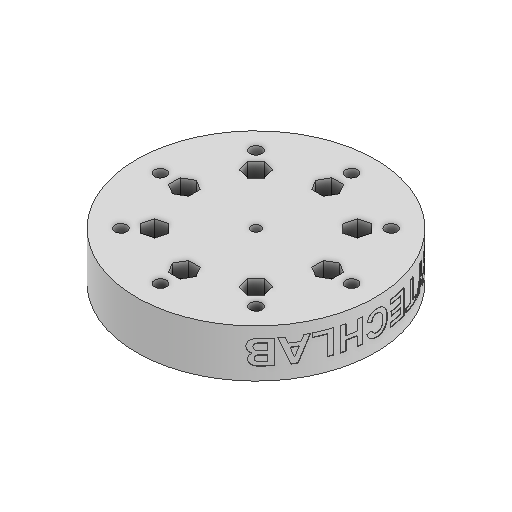
# Autodesk Inventor part: 3DP_ASA_Cone_and_Disc_Mount
Saved by Autodesk Inventor 2026.1 (Build 301233000, 233)
## iProperties
Created: 2025-06-20
Part Number: 3DP_ASA_Cone_and_Disc_Mount
Material: Generic
Document SubType Name: Modeling
Designer: User
Density: 1 g/cm^3
Appearance: Default
Author: User
Autodesk Inventor part; units mm, degrees
ref_plane "XZ Plane" through (0, 0, 0) normal (0, 1, 0) x (-1, 0, 0)
ref_plane "XY Plane" through (0, 0, 0) normal (0, 0, 1) x (1, 0, 0)
sketch "Sketch1" plane through (0, 0, 0) normal (0, 1, 0) x (-1, 0, 0)
  circle A0 centre (0, 0) radius 50
  line L0 (0, 50) -> (0, -50)
  point P0 (0, 40)
  point P1 (-28.2843, 28.2843)
  point P2 (-40, 0)
  point P3 (-28.2843, -28.2843)
  point P4 (0, -40)
  point P5 (28.2843, -28.2843)
  point P6 (40, 0)
  point P7 (28.2843, 28.2843)
  point P8 (0, 30)
  point P9 (-21.2132, 21.2132)
  point P10 (-30, 0)
  point P11 (-21.2132, -21.2132)
  point P12 (0, -30)
  point P13 (21.2132, -21.2132)
  point P14 (30, 0)
  point P15 (21.2132, 21.2132)
  dimension "d0" = 100
  dimension "d1" = 40
  dimension "d4" = 360
  dimension "d15" = 30
  dimension "d18" = 360
  constraints: 2 end point, 2 point on circle, 2 point on line, 1 centre point, 1 coincident, 1 midpoint, 1 vertical, 18 other
  measures "d0" diameter of A0
  measures "d1" distance of point (0, 0) point (0, 40)
  measures "d15" distance of point (0, 0) point (0, 30)
extrude "Extrusion1" add sketch "Sketch1" along normal blind 20
hole "Hole2" at (0, 0, 40) at (28.2843, 0, 28.2843) at (40, 0, 0) at (28.2843, 0, -28.2843) at (0, 0, -40) at (-28.2843, 0, -28.2843) at (-40, 0, 0) at (-28.2843, 0, 28.2843) at (0, 0, 30) at (21.2132, 0, 21.2132) at (30, 0, 0) at (21.2132, 0, -21.2132) at (0, 0, -30) at (-21.2132, 0, -21.2132) at (-30, 0, 0) at (-21.2132, 0, 21.2132) direction (0, 1, 0) diameter 5 end through all
sketch "Sketch2" plane through (0, 20, 0) normal (0, 1, 0) x (1, 0, 0)
  circle A0 centre (-21.2132, -21.2132) radius 2.5 projected
  circle A1 centre (-30, 0) radius 2.5 projected
  circle A2 centre (-21.2132, 21.2132) radius 2.5 projected
  circle A3 centre (0, 30) radius 2.5 projected
  circle A4 centre (21.2132, 21.2132) radius 2.5 projected
  circle A5 centre (30, 0) radius 2.5 projected
  circle A6 centre (21.2132, -21.2132) radius 2.5 projected
  circle A7 centre (0, -30) radius 2.5 projected
  circle A8 centre (-28.2843, -28.2843) radius 2.5 projected
  circle A9 centre (-40, 0) radius 2.5 projected
  circle A10 centre (-28.2843, 28.2843) radius 2.5 projected
  circle A11 centre (0, 40) radius 2.5 projected
  circle A12 centre (28.2843, 28.2843) radius 2.5 projected
  circle A13 centre (40, 0) radius 2.5 projected
  circle A14 centre (28.2843, -28.2843) radius 2.5 projected
  circle A15 centre (0, -40) radius 2.5 projected
  circle A16 centre (0, 0) radius 50 projected
  line L0 (-2.4537, -34.25) -> (-4.9075, -30)
  line L1 (-4.9075, -30) -> (-2.4537, -25.75)
  line L2 (-2.4537, -25.75) -> (2.4537, -25.75)
  line L3 (2.4537, -25.75) -> (4.9075, -30)
  line L4 (4.9075, -30) -> (2.4537, -34.25)
  line L5 (2.4537, -34.25) -> (-2.4537, -34.25)
  line L6 (16.4729, -19.9431) -> (19.9431, -16.4729)
  line L7 (19.9431, -16.4729) -> (24.6833, -17.7431)
  line L8 (17.7431, -24.6833) -> (16.4729, -19.9431)
  line L9 (24.6833, -17.7431) -> (25.9535, -22.4834)
  line L10 (25.9535, -22.4834) -> (22.4834, -25.9535)
  line L11 (22.4834, -25.9535) -> (17.7431, -24.6833)
  line L12 (25.75, -2.4537) -> (25.75, 2.4537)
  line L13 (25.75, 2.4537) -> (30, 4.9075)
  line L14 (30, -4.9075) -> (25.75, -2.4537)
  line L15 (30, 4.9075) -> (34.25, 2.4537)
  line L16 (34.25, 2.4537) -> (34.25, -2.4537)
  line L17 (34.25, -2.4537) -> (30, -4.9075)
  line L18 (19.9431, 16.4729) -> (16.4729, 19.9431)
  line L19 (16.4729, 19.9431) -> (17.7431, 24.6833)
  line L20 (24.6833, 17.7431) -> (19.9431, 16.4729)
  line L21 (17.7431, 24.6833) -> (22.4834, 25.9535)
  line L22 (22.4834, 25.9535) -> (25.9535, 22.4834)
  line L23 (25.9535, 22.4834) -> (24.6833, 17.7431)
  line L24 (2.4537, 25.75) -> (-2.4537, 25.75)
  line L25 (-2.4537, 25.75) -> (-4.9075, 30)
  line L26 (4.9075, 30) -> (2.4537, 25.75)
  line L27 (-4.9075, 30) -> (-2.4537, 34.25)
  line L28 (-2.4537, 34.25) -> (2.4537, 34.25)
  line L29 (2.4537, 34.25) -> (4.9075, 30)
  line L30 (-16.4729, 19.9431) -> (-19.9431, 16.4729)
  line L31 (-19.9431, 16.4729) -> (-24.6833, 17.7431)
  line L32 (-17.7431, 24.6833) -> (-16.4729, 19.9431)
  line L33 (-24.6833, 17.7431) -> (-25.9535, 22.4834)
  line L34 (-25.9535, 22.4834) -> (-22.4834, 25.9535)
  line L35 (-22.4834, 25.9535) -> (-17.7431, 24.6833)
  line L36 (-25.75, 2.4537) -> (-25.75, -2.4537)
  line L37 (-25.75, -2.4537) -> (-30, -4.9075)
  line L38 (-30, 4.9075) -> (-25.75, 2.4537)
  line L39 (-30, -4.9075) -> (-34.25, -2.4537)
  line L40 (-34.25, -2.4537) -> (-34.25, 2.4537)
  line L41 (-34.25, 2.4537) -> (-30, 4.9075)
  line L42 (-19.9431, -16.4729) -> (-16.4729, -19.9431)
  line L43 (-16.4729, -19.9431) -> (-17.7431, -24.6833)
  line L44 (-24.6833, -17.7431) -> (-19.9431, -16.4729)
  line L45 (-17.7431, -24.6833) -> (-22.4834, -25.9535)
  line L46 (-22.4834, -25.9535) -> (-25.9535, -22.4834)
  line L47 (-25.9535, -22.4834) -> (-24.6833, -17.7431)
  point P0 (30, 0)
  point P1 (21.2132, 21.2132)
  point P2 (0, 30)
  point P3 (-21.2132, 21.2132)
  point P4 (-30, 0)
  dimension "d27" = 8.5
  dimension "d30" = 360
  constraints: 96 end point, 1 coincident, 118 other
  measures "d27" distance between parallel lines of L2 L5
extrude "Extrusion2" cut sketch "Sketch2" against normal blind 12.5 contours L0 L1 L2 L3 L4 L5 | L6 L7 L9 L10 L11 L8 | L12 L13 L15 L16 L17 L14 | L18 L19 L21 L22 L23 L20 | L24 L25 L27 L28 L29 L26 | L30 L31 L33 L34 L35 L32 | L36 L37 L39 L40 L41 L38 | L42 L43 L45 L46 L47 L44
sketch "Sketch3" plane through (0, 0, 0) normal (0, -1, 0) x (1, 0, 0)
  circle A0 centre (-21.2132, 21.2132) radius 2.5 projected
  circle A1 centre (-30, 0) radius 2.5 projected
  circle A2 centre (-21.2132, -21.2132) radius 2.5 projected
  circle A3 centre (0, -30) radius 2.5 projected
  circle A4 centre (21.2132, -21.2132) radius 2.5 projected
  circle A5 centre (30, 0) radius 2.5 projected
  circle A6 centre (21.2132, 21.2132) radius 2.5 projected
  circle A7 centre (0, 30) radius 2.5 projected
  circle A8 centre (-28.2843, 28.2843) radius 2.5 projected
  circle A9 centre (-40, 0) radius 2.5 projected
  circle A10 centre (-28.2843, -28.2843) radius 2.5 projected
  circle A11 centre (0, -40) radius 2.5 projected
  circle A12 centre (28.2843, -28.2843) radius 2.5 projected
  circle A13 centre (40, 0) radius 2.5 projected
  circle A14 centre (28.2843, 28.2843) radius 2.5 projected
  circle A15 centre (0, 40) radius 2.5 projected
  circle A16 centre (0, 0) radius 50 projected
  line L0 (-35.75, -2.4537) -> (-40, -4.9075)
  line L1 (-40, -4.9075) -> (-44.25, -2.4537)
  line L2 (-44.25, -2.4537) -> (-44.25, 2.4537)
  line L3 (-44.25, 2.4537) -> (-40, 4.9075)
  line L4 (-40, 4.9075) -> (-35.75, 2.4537)
  line L5 (-35.75, 2.4537) -> (-35.75, -2.4537)
  line L6 (-27.0141, -23.544) -> (-23.544, -27.0141)
  line L7 (-31.7544, -24.8142) -> (-27.0141, -23.544)
  line L8 (-33.0245, -29.5544) -> (-31.7544, -24.8142)
  line L9 (-23.544, -27.0141) -> (-24.8142, -31.7544)
  line L10 (-29.5544, -33.0245) -> (-33.0245, -29.5544)
  line L11 (-24.8142, -31.7544) -> (-29.5544, -33.0245)
  line L12 (-2.4537, -35.75) -> (2.4537, -35.75)
  line L13 (-4.9075, -40) -> (-2.4537, -35.75)
  line L14 (-2.4537, -44.25) -> (-4.9075, -40)
  line L15 (2.4537, -35.75) -> (4.9075, -40)
  line L16 (2.4537, -44.25) -> (-2.4537, -44.25)
  line L17 (4.9075, -40) -> (2.4537, -44.25)
  line L18 (23.544, -27.0141) -> (27.0141, -23.544)
  line L19 (24.8142, -31.7544) -> (23.544, -27.0141)
  line L20 (29.5544, -33.0245) -> (24.8142, -31.7544)
  line L21 (27.0141, -23.544) -> (31.7544, -24.8142)
  line L22 (33.0245, -29.5544) -> (29.5544, -33.0245)
  line L23 (31.7544, -24.8142) -> (33.0245, -29.5544)
  line L24 (35.75, -2.4537) -> (35.75, 2.4537)
  line L25 (40, -4.9075) -> (35.75, -2.4537)
  line L26 (44.25, -2.4537) -> (40, -4.9075)
  line L27 (35.75, 2.4537) -> (40, 4.9075)
  line L28 (44.25, 2.4537) -> (44.25, -2.4537)
  line L29 (40, 4.9075) -> (44.25, 2.4537)
  line L30 (27.0141, 23.544) -> (23.544, 27.0141)
  line L31 (31.7544, 24.8142) -> (27.0141, 23.544)
  line L32 (33.0245, 29.5544) -> (31.7544, 24.8142)
  line L33 (23.544, 27.0141) -> (24.8142, 31.7544)
  line L34 (29.5544, 33.0245) -> (33.0245, 29.5544)
  line L35 (24.8142, 31.7544) -> (29.5544, 33.0245)
  line L36 (2.4537, 35.75) -> (-2.4537, 35.75)
  line L37 (4.9075, 40) -> (2.4537, 35.75)
  line L38 (2.4537, 44.25) -> (4.9075, 40)
  line L39 (-2.4537, 35.75) -> (-4.9075, 40)
  line L40 (-2.4537, 44.25) -> (2.4537, 44.25)
  line L41 (-4.9075, 40) -> (-2.4537, 44.25)
  line L42 (-23.544, 27.0141) -> (-27.0141, 23.544)
  line L43 (-24.8142, 31.7544) -> (-23.544, 27.0141)
  line L44 (-29.5544, 33.0245) -> (-24.8142, 31.7544)
  line L45 (-27.0141, 23.544) -> (-31.7544, 24.8142)
  line L46 (-33.0245, 29.5544) -> (-29.5544, 33.0245)
  line L47 (-31.7544, 24.8142) -> (-33.0245, 29.5544)
  point P0 (0, -40)
  point P1 (-28.2843, 28.2843)
  dimension "d34" = 8.5
  dimension "d37" = 360
  constraints: 96 end point, 1 coincident, 118 other
  measures "d34" distance between parallel lines of L2 L5
extrude "Extrusion3" cut sketch "Sketch3" against normal blind 12.5 contours A8 | A10 | L0 L1 L2 L3 L4 L5 | L6 L9 L11 L10 L8 L7 | L12 L15 L17 L16 L14 L13 | L18 L21 L23 L22 L20 L19 | L24 L27 L29 L28 L26 L25 | L30 L33 L35 L34 L32 L31 | L36 L39 L41 L40 L38 L37 | L42 L45 L47 L46 L44 L43
ref_plane "Work Plane1" through (50, 0, 0) normal (1, 0, 0) x (0, 1, 0)
sketch "Sketch4" plane through (50, 0, 0) normal (1, 0, 0) x (0, 1, 0)
  line L0 (5.2475, -38.8454) -> (5.2475, 38.603) construction
  line L1 (5.2475, 38.603) -> (21.5172, 38.603) construction
  line L2 (21.5172, 38.603) -> (21.5172, -38.8454) construction
  line L3 (21.5172, -38.8454) -> (5.2475, -38.8454) construction
  line L4 (5.4152, -42.1867) -> (5.4152, -38.1852)
  spline S0 degree 2 poles (5.4152, -38.1852) (5.4152, -36.9962) (5.6134, -35.83) (6.2384, -34.9078) (7.2826, -34.2904) (7.9304, -34.2904) knots 0 0 0 1 2 3 4 4 4
  spline S1 degree 2 poles (7.9304, -34.2904) (8.6316, -34.2904) (9.7978, -35.045) (10.0951, -35.6928) knots 0 0 0 1 2 2 2
  spline S2 degree 2 poles (10.0951, -35.6928) (10.3618, -34.7782) (11.6423, -33.8026) (12.5112, -33.8026) knots 0 0 0 1 2 2 2
  spline S3 degree 2 poles (12.5112, -33.8026) (13.1972, -33.8026) (14.4853, -34.4352) (15.2551, -35.5404) (15.3466, -36.3407) knots 0 0 0 1 2 3 3 3
  spline S4 degree 2 poles (15.3466, -36.3407) (15.3999, -36.8514) (15.4152, -38.7797) knots 0 0 0 1 1 1
  line L5 (15.4152, -38.7797) -> (15.4152, -42.1867)
  line L6 (15.4152, -42.1867) -> (5.4152, -42.1867)
  line L7 (11.0478, -40.1669) -> (13.7231, -40.1669)
  line L8 (13.7231, -40.1669) -> (13.7231, -38.2919)
  spline S5 degree 2 poles (13.7231, -38.2919) (13.7231, -37.1944) (13.6621, -36.9047) knots 0 0 0 1 1 1
  spline S6 degree 2 poles (13.6621, -36.9047) (13.5783, -36.455) (12.9457, -35.8834) (12.4121, -35.8834) knots 0 0 0 1 2 2 2
  spline S7 degree 2 poles (12.4121, -35.8834) (11.9624, -35.8834) (11.3374, -36.3178) (11.0478, -37.1486) (11.0478, -38.5282) knots 0 0 0 1 2 3 3 3
  line L9 (11.0478, -38.5282) -> (11.0478, -40.1669)
  line L10 (7.0768, -40.1669) -> (9.3862, -40.1669)
  line L11 (9.3862, -40.1669) -> (9.3862, -38.8407)
  spline S8 degree 2 poles (9.3862, -38.8407) (9.3862, -37.6593) (9.3557, -37.3697) knots 0 0 0 1 1 1
  spline S9 degree 2 poles (9.3557, -37.3697) (9.2871, -36.8514) (8.7002, -36.2569) (8.2124, -36.2569) knots 0 0 0 1 2 2 2
  spline S10 degree 2 poles (8.2124, -36.2569) (7.7475, -36.2569) (7.1759, -36.7675) (7.1073, -37.2782) knots 0 0 0 1 2 2 2
  spline S11 degree 2 poles (7.1073, -37.2782) (7.0768, -37.5755) (7.0768, -39.0084) knots 0 0 0 1 1 1
  line L12 (7.0768, -39.0084) -> (7.0768, -40.1669)
  line L13 (15.4152, -29.4733) -> (11.2079, -29.4733)
  line L14 (11.2079, -29.4733) -> (5.4152, -33.1319)
  line L15 (5.4152, -33.1319) -> (5.4152, -30.7691)
  line L16 (5.4152, -30.7691) -> (9.3786, -28.4062)
  line L17 (9.3786, -28.4062) -> (5.4152, -26.1044)
  line L18 (5.4152, -26.1044) -> (5.4152, -23.7721)
  line L19 (5.4152, -23.7721) -> (11.2231, -27.4535)
  line L20 (11.2231, -27.4535) -> (15.4152, -27.4535)
  line L21 (15.4152, -27.4535) -> (15.4152, -29.4733)
  line L22 (15.4152, -20.5251) -> (7.1073, -20.5251)
  line L23 (7.1073, -20.5251) -> (7.1073, -23.4901)
  line L24 (7.1073, -23.4901) -> (5.4152, -23.4901)
  line L25 (5.4152, -23.4901) -> (5.4152, -15.548)
  line L26 (5.4152, -15.548) -> (7.1073, -15.548)
  line L27 (7.1073, -15.548) -> (7.1073, -18.5053)
  line L28 (7.1073, -18.5053) -> (15.4152, -18.5053)
  line L29 (15.4152, -18.5053) -> (15.4152, -20.5251)
  line L30 (15.4152, -14.237) -> (5.4152, -14.237)
  line L31 (5.4152, -14.237) -> (5.4152, -6.8209)
  line L32 (5.4152, -6.8209) -> (7.1073, -6.8209)
  line L33 (7.1073, -6.8209) -> (7.1073, -12.2172)
  line L34 (7.1073, -12.2172) -> (9.3252, -12.2172)
  line L35 (9.3252, -12.2172) -> (9.3252, -7.1944)
  line L36 (9.3252, -7.1944) -> (11.0173, -7.1944)
  line L37 (11.0173, -7.1944) -> (11.0173, -12.2172)
  line L38 (11.0173, -12.2172) -> (13.7231, -12.2172)
  line L39 (13.7231, -12.2172) -> (13.7231, -6.6303)
  line L40 (13.7231, -6.6303) -> (15.4152, -6.6303)
  line L41 (15.4152, -6.6303) -> (15.4152, -14.237)
  line L42 (11.7338, 1.4794) -> (12.3512, 3.4383)
  spline S12 degree 2 poles (12.3512, 3.4383) (13.9899, 2.9886) (15.5829, 0.8925) (15.5829, -0.7157) knots 0 0 0 1 2 2 2
  spline S13 degree 2 poles (15.5829, -0.7157) (15.5829, -2.705) (12.8618, -5.2736) (10.5066, -5.2736) knots 0 0 0 1 2 2 2
  spline S14 degree 2 poles (10.5066, -5.2736) (8.0066, -5.2736) (5.2475, -2.6974) (5.2475, -0.5937) knots 0 0 0 1 2 2 2
  spline S15 degree 2 poles (5.2475, -0.5937) (5.2475, 1.2355) (6.3298, 2.3864) knots 0 0 0 1 1 1
  spline S16 degree 2 poles (6.3298, 2.3864) (6.9701, 3.0648) (8.1667, 3.4078) knots 0 0 0 1 1 1
  line L43 (8.1667, 3.4078) -> (8.6469, 1.4108)
  spline S17 degree 2 poles (8.6469, 1.4108) (7.8694, 1.2355) (6.9701, 0.1075) (6.9701, -0.6928) knots 0 0 0 1 2 2 2
  spline S18 degree 2 poles (6.9701, -0.6928) (6.9701, -1.8056) (8.563, -3.1928) (10.3542, -3.1928) knots 0 0 0 1 2 2 2
  spline S19 degree 2 poles (10.3542, -3.1928) (12.2521, -3.1928) (13.8603, -1.8285) (13.8603, -0.7386) knots 0 0 0 1 2 2 2
  spline S20 degree 2 poles (13.8603, -0.7386) (13.8603, 0.0694) (12.8313, 1.2279) (11.7338, 1.4794) knots 0 0 0 1 2 2 2
  line L44 (15.4152, 5.1761) -> (5.4152, 5.1761)
  line L45 (5.4152, 5.1761) -> (5.4152, 7.1959)
  line L46 (5.4152, 7.1959) -> (9.3481, 7.1959)
  line L47 (9.3481, 7.1959) -> (9.3481, 11.1517)
  line L48 (9.3481, 11.1517) -> (5.4152, 11.1517)
  line L49 (5.4152, 11.1517) -> (5.4152, 13.1715)
  line L50 (5.4152, 13.1715) -> (15.4152, 13.1715)
  line L51 (15.4152, 13.1715) -> (15.4152, 11.1517)
  line L52 (15.4152, 11.1517) -> (11.0402, 11.1517)
  line L53 (11.0402, 11.1517) -> (11.0402, 7.1959)
  line L54 (11.0402, 7.1959) -> (15.4152, 7.1959)
  line L55 (15.4152, 7.1959) -> (15.4152, 5.1761)
  line L56 (15.4152, 15.3209) -> (5.499, 15.3209)
  line L57 (5.499, 15.3209) -> (5.499, 17.3407)
  line L58 (5.499, 17.3407) -> (13.7231, 17.3407)
  line L59 (13.7231, 17.3407) -> (13.7231, 22.3636)
  line L60 (13.7231, 22.3636) -> (15.4152, 22.3636)
  line L61 (15.4152, 22.3636) -> (15.4152, 15.3209)
  line L62 (15.4152, 32.8133) -> (15.4152, 30.6181)
  line L63 (15.4152, 30.6181) -> (13.1438, 29.7492)
  line L64 (13.1438, 29.7492) -> (13.1438, 25.7553)
  line L65 (13.1438, 25.7553) -> (15.4152, 24.9245)
  line L66 (15.4152, 24.9245) -> (15.4152, 22.7828)
  line L67 (15.4152, 22.7828) -> (5.4152, 26.67)
  line L68 (5.4152, 26.67) -> (5.4152, 28.8194)
  line L69 (5.4152, 28.8194) -> (15.4152, 32.8133)
  line L70 (11.4518, 29.1014) -> (7.7475, 27.7218)
  line L71 (7.7475, 27.7218) -> (11.4518, 26.3651)
  line L72 (11.4518, 26.3651) -> (11.4518, 29.1014)
  line L73 (5.4152, 33.8956) -> (5.4152, 37.8971)
  spline S21 degree 2 poles (5.4152, 37.8971) (5.4152, 39.0861) (5.6134, 40.2523) (6.2384, 41.1745) (7.2826, 41.7919) (7.9304, 41.7919) knots 0 0 0 1 2 3 4 4 4
  spline S22 degree 2 poles (7.9304, 41.7919) (8.6316, 41.7919) (9.7978, 41.0374) (10.0951, 40.3895) knots 0 0 0 1 2 2 2
  spline S23 degree 2 poles (10.0951, 40.3895) (10.3618, 41.3041) (11.6423, 42.2797) (12.5112, 42.2797) knots 0 0 0 1 2 2 2
  spline S24 degree 2 poles (12.5112, 42.2797) (13.1972, 42.2797) (14.4853, 41.6471) (15.2551, 40.5419) (15.3466, 39.7416) knots 0 0 0 1 2 3 3 3
  spline S25 degree 2 poles (15.3466, 39.7416) (15.3999, 39.2309) (15.4152, 37.3026) knots 0 0 0 1 1 1
  line L74 (15.4152, 37.3026) -> (15.4152, 33.8956)
  line L75 (15.4152, 33.8956) -> (5.4152, 33.8956)
  line L76 (11.0478, 35.9154) -> (13.7231, 35.9154)
  line L77 (13.7231, 35.9154) -> (13.7231, 37.7904)
  spline S26 degree 2 poles (13.7231, 37.7904) (13.7231, 38.888) (13.6621, 39.1776) knots 0 0 0 1 1 1
  spline S27 degree 2 poles (13.6621, 39.1776) (13.5783, 39.6273) (12.9457, 40.1989) (12.4121, 40.1989) knots 0 0 0 1 2 2 2
  spline S28 degree 2 poles (12.4121, 40.1989) (11.9624, 40.1989) (11.3374, 39.7645) (11.0478, 38.9337) (11.0478, 37.5541) knots 0 0 0 1 2 3 3 3
  line L78 (11.0478, 37.5541) -> (11.0478, 35.9154)
  line L79 (7.0768, 35.9154) -> (9.3862, 35.9154)
  line L80 (9.3862, 35.9154) -> (9.3862, 37.2416)
  spline S29 degree 2 poles (9.3862, 37.2416) (9.3862, 38.423) (9.3557, 38.7127) knots 0 0 0 1 1 1
  spline S30 degree 2 poles (9.3557, 38.7127) (9.2871, 39.2309) (8.7002, 39.8255) (8.2124, 39.8255) knots 0 0 0 1 2 2 2
  spline S31 degree 2 poles (8.2124, 39.8255) (7.7475, 39.8255) (7.1759, 39.3148) (7.1073, 38.8041) knots 0 0 0 1 2 2 2
  spline S32 degree 2 poles (7.1073, 38.8041) (7.0768, 38.5069) (7.0768, 37.0739) knots 0 0 0 1 1 1
  line L81 (7.0768, 37.0739) -> (7.0768, 35.9154)
  point P0 (0, 0)
  constraints: 2 other
emboss "Emboss1" sketch "Sketch4" operation cut depth 0.2 direction (1, 0, 0) wrap yes faces at (32.9673, 13.3333, 37.592)
sketch "Sketch5" plane through (0, 0, 0) normal (0, -1, 0) x (1, 0, 0)
  circle A0 centre (0, 0) radius 2
  dimension "d44" = 4
  constraints: 1 centre point, 1 coincident
  measures "d44" diameter of A0
extrude "Extrusion4" cut sketch "Sketch5" against normal through all
body "Solid1"
